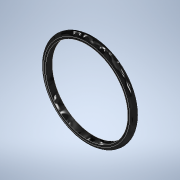
# Autodesk Inventor part: tamiya-slim-tire-gomu
Saved by Autodesk Inventor 2021 (Build 250183000, 183)
## iProperties
Created: 2023-10-14
Part Number: tamiya-slim-tire-gomu
Material: 一般
Document SubType Name: Modeling
Designer: takag
Density: 1 g/cm^3
Appearance: 黒
Author: takag
Autodesk Inventor part; units mm, degrees
ref_plane "YZ Plane" through (0, 0, 0) normal (1, 0, 0) x (0, 1, 0)
ref_plane "XZ Plane" through (0, 0, 0) normal (0, 1, 0) x (-1, 0, 0)
ref_plane "XY Plane" through (0, 0, 0) normal (0, 0, 1) x (1, 0, 0)
sketch "スケッチ1" plane through (0, 0, 0) normal (1, 0, 0) x (0, 1, 0)
  line L0 (24.3, 0) -> (24.3, 2)
  line L1 (24.3, 0) -> (24.3, -2)
  circle A0 centre (25.5, 0) radius 2
  line L2 (24.3, 2) -> (25.5, 2)
  line L3 (24.3, -2) -> (25.5, -2)
  line L4 (0, 0) -> (0, -5)
  point P0 (27.5, 0)
  dimension "d0" = 2
  dimension "d1" = 2
  dimension "d2" = 24.3
  dimension "d3" = 27.5
  dimension "d4" = 4
  dimension "d5" = 5
  constraints: 10 end point, 3 point on circle, 3 vertical, 2 tangent, 1 centre point
  measures "d0" distance of L0.start L0.end
  measures "d1" distance of L0.start L1.end
  measures "d2" distance of L4.start L0.start
  measures "d3" distance of L4.start A0.start
  measures "d4" diameter of A0
  measures "d5" distance of L4.start L4.end
revolve "回転1" add sketch "スケッチ1" angle 360 about axis through (0, 0, 0) along (0, 0, -1) picked at (26.4166, -0.1483) contours L0 A0 L1 | L0 L2 A0 | A0 L3 L1
